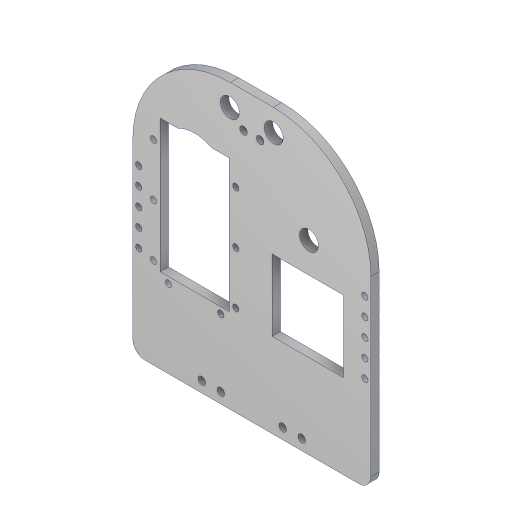
# Autodesk Inventor part: Box_Front
Saved by Autodesk Inventor 2023.2 (Build 272271000, 271)
## iProperties
Created: 2021-07-28
Part Number: Box_Front
Material: 알루미늄 6061
Document SubType Name: Modeling
Designer: user
Density: 2.7 g/cm^3
Appearance: 알루미늄 - 평지
Mass: 86.6795 g
Surface Area: 213.653 cm^2
Volume: 32.1035 cm^3
Author: user
Autodesk Inventor part; units mm, degrees
ref_plane "YZ Plane" through (0, 0, 0) normal (1, 0, 0) x (0, 1, 0)
ref_plane "XZ Plane" through (0, 0, 0) normal (0, 1, 0) x (-1, 0, 0)
ref_plane "XY Plane" through (0, 0, 0) normal (0, 0, 1) x (1, 0, 0)
sketch "스케치1" plane through (0, 0, 0) normal (0, 0, 1) x (1, 0, 0)
  line L0 (-50.01, 54) -> (50.01, 54)
  line L1 (50.01, 54) -> (50.01, -40)
  line L2 (50.01, -40) -> (-50.01, -40)
  line L3 (-50.01, -40) -> (-50.01, 54)
  point P0 (0, 0)
  dimension "d0" = 100.02
  dimension "d1" = 50.01
  dimension "d2" = 94
  dimension "d3" = 40
  constraints: 8 end point, 2 parallel, 1 horizontal, 1 perpendicular
  measures "d0" distance of L1.end L2.end
  measures "d1" distance from line of L3 point (0, 0)
  measures "d2" distance between parallel lines of L2 L0
  measures "d3" distance from line of L2 point (0, 0)
extrude "돌출1" add sketch "스케치1" along normal blind 3.5
sketch "스케치2" plane through (0, 0, 3.5) normal (0, 0, 1) x (1, 0, 0)
  circle A0 centre (-24.01, 13.1) radius 14
  line L0 (-50.01, -40) -> (50.01, -40) projected
  point P0 (0, 0)
  dimension "d6" = 28
  dimension "d7" = 24.01
  dimension "d8" = 53.1
  constraints: 1 centre point
  measures "d6" diameter of A0
  measures "d7" horizontal distance of point (0, 0) A0.centre
  measures "d8" distance from line of L0 A0.centre
extrude "돌출2" cut sketch "스케치2" against normal up to surface (3.5 mm away)
sketch "스케치3" plane through (0, 0, 3.5) normal (0, 0, 1) x (1, 0, 0)
  line L0 (-9.49, -29.6) -> (-38.53, -29.6)
  line L1 (-38.53, -29.6) -> (-38.53, 26.3)
  line L2 (-38.53, 26.3) -> (-9.49, 26.3)
  line L3 (-9.49, 26.3) -> (-9.49, -29.6)
  line L4 (-50.01, -40) -> (50.01, -40) projected
  circle A0 centre (-24.01, 13.1) radius 14 projected
  point P0 (0, 0)
  dimension "d11" = 10.4
  dimension "d12" = 55.9
  dimension "d13" = 29.04
  dimension "d14" = 14.52
  constraints: 8 end point, 2 parallel, 1 horizontal, 1 perpendicular
  measures "d11" distance between parallel lines of L4 L0
  measures "d12" distance between parallel lines of L0 L2
  measures "d13" distance between parallel lines of L3 L1
  measures "d14" distance from line of L1 A0.centre
extrude "돌출3" cut sketch "스케치3" against normal up to surface (3.5 mm away) contours L0 L1 L2 A0 L3 | A0 L2 picked at (-19.646, 17.031)
sketch "스케치4" plane through (0, 0, 3.5) normal (0, 0, 1) x (1, 0, 0)
  line L0 (-38.53, -29.6) -> (-38.53, 26.3) projected
  line L1 (-9.49, 26.3) -> (-9.49, -29.6) projected
  line L2 (-9.49, -29.6) -> (-38.53, -29.6) projected
  arc A0 (-19.3452, 26.3) -> (-28.6748, 26.3) centre (-24.01, 13.1) ccw projected
  arc A1 (-16.8854, 26.3) -> (-31.1346, 26.3) centre (-24.01, 13.1) ccw
  line L3 (-38.53, 26.3) -> (-28.6748, 26.3) projected
  line L4 (-19.3452, 26.3) -> (-9.49, 26.3) projected
  point P0 (0, 0)
  constraints: 2 point on circle, 2 point on line, 1 centre point, 1 coincident
extrude "돌출4" cut sketch "스케치4" against normal up to surface (3.5 mm away)
sketch "스케치5" plane through (0, 0, 3.5) normal (0, 0, 1) x (1, 0, 0)
  arc A0 (-16.8854, 26.3) -> (-31.1346, 26.3) centre (-24.01, 13.1) ccw projected
  circle A1 centre (-24.01, 13.1) radius 5
  circle A2 centre (-6.71, -4.9) radius 1.705
  circle A3 centre (-6.71, 17.1) radius 1.705
  circle A4 centre (-6.71, -26.9) radius 1.7
  circle A5 centre (-13.01, -32.2) radius 1.705
  circle A6 centre (-35.01, -32.2) radius 1.705
  circle A7 centre (-41.31, -26.9) radius 1.705
  circle A8 centre (-41.31, -4.9) radius 1.705
  circle A9 centre (-41.31, 17.1) radius 1.705
  circle A10 centre (-41.31, 17.1) radius 1.35
  circle A11 centre (-41.31, -4.9) radius 1.35
  circle A12 centre (-41.31, -26.9) radius 1.35
  circle A13 centre (-35.01, -32.2) radius 1.35
  circle A14 centre (-13.01, -32.2) radius 1.35
  circle A15 centre (-6.71, -26.9) radius 1.35
  circle A16 centre (-6.71, -4.9) radius 1.35
  circle A17 centre (-6.71, 17.1) radius 1.35
  point P0 (0, 0)
  dimension "d20" = 3.41
  dimension "d21" = 2.7
  dimension "d22" = 2.7
  dimension "d23" = 2.7
  dimension "d24" = 2.7
  dimension "d25" = 2.7
  dimension "d26" = 2.7
  dimension "d27" = 2.7
  dimension "d28" = 2.7
  constraints: 17 centre point, 8 coincident
  measures "d20" diameter of A9
  measures "d21" diameter of A10
  measures "d22" diameter of A11
  measures "d23" diameter of A12
  measures "d24" diameter of A13
  measures "d25" diameter of A14
  measures "d26" diameter of A15
  measures "d27" diameter of A16
  measures "d28" diameter of A17
extrude "돌출5" cut sketch "스케치5" against normal up to surface (3.5 mm away) contours A10 | A11 | A12 | A13 | A14 | A15 | A16 | A17
sketch "스케치6" plane through (0, 0, 3.5) normal (0, 0, 1) x (1, 0, 0)
  arc A0 (-16.8854, 26.3) -> (-31.1346, 26.3) centre (-24.01, 13.1) ccw projected
  line L0 (-24.01, 13.1) -> (24.01, 13.1)
  line L1 (-24.01, 13.1) -> (24.01, 13.1) construction
  circle A1 centre (24.01, 13.1) radius 4.025
  point P0 (0, 0)
  dimension "d31" = 48.02
  dimension "d32" = 0
  dimension "d33" = 8.05
  constraints: 4 end point, 2 horizontal, 1 centre point, 1 coincident, 1 collinear
  measures "d31" distance of L0.start L0.end
  measures "d32" distance between parallel lines of L0 L1
  measures "d33" diameter of A1
extrude "돌출6" cut sketch "스케치6" against normal up to surface (3.5 mm away)
chamfer "모따기2" distance 1.25 angle 45 8 edges at (-8.06, 17.1, 0) (-8.06, -4.9, 0) (-8.06, -26.9, 0) (-14.36, -32.2, 0) (-36.36, -32.2, 0) (-42.66, -26.9, 0) (-42.66, -4.9, 0) (-42.66, 17.1, 0)
sketch "스케치7" plane through (0, 0, 0) normal (0, 0, -1) x (-1, 0, 0)
  arc A0 (31.1346, 26.3) -> (16.8854, 26.3) centre (24.01, 13.1) ccw projected
  line L0 (24.01, 13.1) -> (9.2184, 44.8208)
  line L1 (24.01, 13.1) -> (59.01, 13.1) construction
  circle A1 centre (9.2184, 44.8208) radius 4.025
  circle A2 centre (-24.01, 13.1) radius 4.025 projected
  line L2 (-24.01, 13.1) -> (-9.2184, 44.8208)
  line L3 (-24.01, 13.1) -> (10.99, 13.1) construction
  circle A3 centre (-9.2184, 44.8208) radius 4.025
  point P0 (0, 0)
  dimension "d42" = 35
  dimension "d43" = 115
  dimension "d44" = 8.05
  dimension "d45" = 35
  dimension "d46" = 65
  dimension "d47" = 8.05
  constraints: 8 end point, 2 centre point, 2 coincident, 2 equal length, 2 horizontal
  measures "d42" distance of L0.start L0.end
  measures "d43" angle of L1 L0
  measures "d44" diameter of A1
  measures "d45" distance of L2.start L2.end
  measures "d46" angle of L3 L2
  measures "d47" diameter of A3
extrude "돌출7" cut sketch "스케치7" against normal up to surface (3.5 mm away) contours A1 | A3
fillet "모깎기1" radius 41 2 edges at (-50.01, 54, 1.75) (50.01, 54, 1.75)
sketch "스케치8" plane through (0, 0, 0) normal (0, 0, -1) x (-1, 0, 0)
  circle A0 centre (-47.51, -25.5) radius 1.35
  circle A1 centre (-47.51, -18) radius 1.35
  circle A2 centre (-47.51, -10.5) radius 1.35
  circle A3 centre (-47.51, -3) radius 1.35
  circle A4 centre (-47.51, 4.5) radius 1.35
  line L0 (-50.01, 13) -> (-50.01, -40) projected
  line L1 (-50.01, -40) -> (50.01, -40) projected
  point P0 (0, 0)
  dimension "d51" = 2.7
  dimension "d52" = 2.7
  dimension "d53" = 2.7
  dimension "d54" = 2.7
  dimension "d55" = 2.7
  dimension "d56" = 2.5
  dimension "d57" = 2.5
  dimension "d58" = 2.5
  dimension "d59" = 2.5
  dimension "d60" = 2.5
  dimension "d61" = 14.5
  dimension "d62" = 7.5
  dimension "d63" = 15
  dimension "d64" = 22.5
  dimension "d65" = 30
  constraints: 5 centre point
  measures "d51" diameter of A0
  measures "d52" diameter of A1
  measures "d53" diameter of A2
  measures "d54" diameter of A3
  measures "d55" diameter of A4
  measures "d56" distance from line of L0 A0.centre
  measures "d57" distance from line of L0 A1.centre
  measures "d58" distance from line of L0 A2.centre
  measures "d59" distance from line of L0 A3.centre
  measures "d60" distance from line of L0 A4.centre
  measures "d61" distance from line of A0.centre L1
  measures "d62" distance of A1.centre A0.centre
  measures "d63" distance of A2.centre A0.centre
  measures "d64" distance of A3.centre A0.centre
  measures "d65" distance of A4.centre A0.centre
extrude "돌출8" cut sketch "스케치8" against normal up to surface (3.5 mm away)
chamfer "모따기3" distance 1.25 angle 45 5 edges at (48.86, -25.5, 0) (48.86, -18, 0) (48.86, -10.5, 0) (48.86, -3, 0) (48.86, 4.5, 0)
sketch "스케치9" plane through (0, 0, 3.5) normal (0, 0, 1) x (1, 0, 0)
  circle A0 centre (-47.51, -25.5) radius 1.35
  circle A1 centre (-47.51, -18) radius 1.35
  circle A2 centre (-47.51, -10.5) radius 1.35
  circle A3 centre (-47.51, -3) radius 1.35
  circle A4 centre (-47.51, 4.5) radius 1.35
  line L0 (-50.01, 13) -> (-50.01, -40) projected
  line L1 (-50.01, -40) -> (50.01, -40) projected
  point P0 (0, 0)
  dimension "d71" = 2.7
  dimension "d72" = 2.7
  dimension "d73" = 2.7
  dimension "d74" = 2.7
  dimension "d75" = 2.7
  dimension "d76" = 2.5
  dimension "d77" = 2.5
  dimension "d78" = 2.5
  dimension "d79" = 2.5
  dimension "d80" = 2.5
  dimension "d81" = 14.5
  dimension "d82" = 22
  dimension "d83" = 29.5
  dimension "d84" = 37
  dimension "d85" = 44.5
  constraints: 5 centre point
  measures "d71" diameter of A0
  measures "d72" diameter of A1
  measures "d73" diameter of A2
  measures "d74" diameter of A3
  measures "d75" diameter of A4
  measures "d76" distance from line of L0 A4.centre
  measures "d77" distance from line of L0 A3.centre
  measures "d78" distance from line of L0 A2.centre
  measures "d79" distance from line of L0 A1.centre
  measures "d80" distance from line of L0 A0.centre
  measures "d81" distance from line of L1 A0.centre
  measures "d82" distance from line of L1 A1.centre
  measures "d83" distance from line of L1 A2.centre
  measures "d84" distance from line of L1 A3.centre
  measures "d85" distance from line of L1 A4.centre
extrude "돌출9" cut sketch "스케치9" against normal up to surface (3.5 mm away)
chamfer "모따기4" distance 1.25 angle 45 5 edges at (-48.86, 4.5, 0) (-48.86, -3, 0) (-48.86, -10.5, 0) (-48.86, -18, 0) (-48.86, -25.5, 0)
sketch "스케치10" plane through (0, 0, 0) normal (0, 0, -1) x (-1, 0, 0)
  line L0 (-50.01, -26.2141) -> (-50.01, -40) projected
  line L1 (50.01, -40) -> (50.01, -26.2141) projected
  line L2 (-50.01, -40) -> (50.01, -40) projected
  line L3 (-50.01, -40) -> (50.01, -40)
  line L4 (50.01, -40) -> (50.01, -65)
  line L5 (50.01, -65) -> (-50.01, -65)
  line L6 (-50.01, -65) -> (-50.01, -40)
  point P0 (0, 0)
  dimension "d100" = 25
  constraints: 8 end point, 2 parallel, 1 horizontal, 1 perpendicular
  measures "d100" distance of L3.end L4.end
extrude "돌출10" add sketch "스케치10" against normal up to surface (3.5 mm away)
sketch "스케치11" plane through (0, 0, 0) normal (0, 0, -1) x (-1, 0, 0)
  line L0 (-25, -58) -> (25, -58)
  line L1 (25, -58) -> (25, -63)
  line L2 (25, -63) -> (-25, -63)
  line L3 (-25, -63) -> (-25, -58)
  line L4 (50.01, -65) -> (-50.01, -65) projected
  circle A0 centre (-21, -60.5) radius 1.6
  circle A1 centre (-13, -60.5) radius 1.6
  circle A2 centre (13, -60.5) radius 1.6
  circle A3 centre (21, -60.5) radius 1.6
  point P0 (0, 0)
  dimension "d103" = 50
  dimension "d104" = 5
  dimension "d105" = 7
  dimension "d106" = 25
  dimension "d107" = 3.2
  dimension "d108" = 3.2
  dimension "d109" = 3.2
  dimension "d110" = 3.2
  dimension "d111" = 2.5
  dimension "d112" = 2.5
  dimension "d113" = 2.5
  dimension "d114" = 2.5
  dimension "d115" = 4
  dimension "d116" = 12
  dimension "d117" = 4
  dimension "d118" = 12
  constraints: 8 end point, 4 centre point, 2 parallel, 1 horizontal, 1 perpendicular
  measures "d103" distance of L1.end L2.end
  measures "d104" distance of L0.end L1.end
  measures "d105" distance between parallel lines of L4 L0
  measures "d106" distance from line of point (0, 0) L1
  measures "d107" diameter of A0
  measures "d108" diameter of A1
  measures "d109" diameter of A2
  measures "d110" diameter of A3
  measures "d111" distance from line of L2 A0.centre
  measures "d112" distance from line of L2 A1.centre
  measures "d113" distance from line of L2 A2.centre
  measures "d114" distance from line of L2 A3.centre
  measures "d115" distance from line of L3 A0.centre
  measures "d116" distance from line of L3 A1.centre
  measures "d117" distance from line of L1 A3.centre
  measures "d118" distance from line of L1 A2.centre
extrude "돌출11" cut sketch "스케치11" against normal up to surface (3.5 mm away) contours A0 | A1 | A2 | A3
fillet "모깎기2" radius 5 2 edges at (50.01, -65, 1.75) (-50.01, -65, 1.75)
sketch "스케치13" plane through (0, 0, 0) normal (0, 0, -1) x (-1, 0, 0)
  line L0 (9.49, 26.3) -> (16.8854, 26.3) projected
  line L1 (16.9, 29.3) -> (-16.9, 29.3)
  line L2 (16.9, 29.3) -> (50.7, 29.3) construction
  line L3 (9.01, 54) -> (-9.01, 54) projected
  line L4 (7, 36.3) -> (-7, 36.3)
  line L5 (-7, 36.3) -> (-7, 39.3)
  line L6 (-4, 42.3) -> (4, 42.3)
  line L7 (7, 39.3) -> (7, 36.3)
  circle A0 centre (3.5, 39.3) radius 1.6
  circle A1 centre (-3.5, 39.3) radius 1.6
  arc A2 (7, 39.3) -> (4, 42.3) centre (4, 39.3) ccw
  arc A3 (-4, 42.3) -> (-7, 39.3) centre (-4, 39.3) ccw
  point P0 (0, 0)
  point P1 (-7, 42.3)
  point P2 (7, 42.3)
  dimension "d149" = 33.8
  dimension "d150" = 180
  dimension "d151" = 16.9
  dimension "d153" = 14
  dimension "d154" = 6
  dimension "d155" = 13
  dimension "d156" = 7
  dimension "d157" = 3.2
  dimension "d158" = 3.2
  dimension "d159" = 3.5
  dimension "d160" = 3.5
  dimension "d161" = 3
  dimension "d162" = 3
  dimension "d169" = 3
  dimension "d170" = 3
  constraints: 12 end point, 4 centre point, 4 point on circle, 4 point on line, 4 tangent, 3 horizontal, 3 parallel, 1 collinear, 1 equal radius, 1 perpendicular
  measures "d149" distance of L1.start L1.end
  measures "d150" angle of L1 L2
  measures "d151" horizontal distance of L1.end point (0, 0)
  measures "d153" distance of point (-7, 42.3) point (7, 42.3)
  measures "d154" distance of L4.end point (-7, 42.3)
  measures "d155" distance between parallel lines of L6 L1
  measures "d156" distance from line of L7 point (0, 0)
  measures "d157" diameter of A0
  measures "d158" diameter of A1
  measures "d159" distance from line of L5 A1.centre
  measures "d160" distance from line of L7 A0.centre
  measures "d161" distance from line of L6 A0.centre
  measures "d162" distance from line of L6 A1.centre
  measures "d169" distance between parallel lines of L1 L0
  measures "d170" radius of A2
extrude "돌출13" cut sketch "스케치13" against normal up to surface (3.5 mm away) contours A0 | A1
chamfer "모따기6" distance 1.5 angle 45 2 edges at (-1.9, 39.3, 0) (5.1, 39.3, 0)
sketch "스케치17" plane through (0, 0, 0) normal (0, 0, -1) x (-1, 0, 0)
  line L0 (-8.51, 0.4) -> (-38.51, 0.4)
  line L1 (-38.51, 0.4) -> (-38.51, -29.6)
  line L2 (-38.51, -29.6) -> (-8.51, -29.6)
  line L3 (-8.51, -29.6) -> (-8.51, 0.4)
  line L4 (-8.51, 0.4) -> (-38.51, -29.6) construction
  line L5 (-38.51, 0.4) -> (-8.51, -29.6) construction
  line L6 (-50.01, -26.2141) -> (-50.01, -60) projected
  line L7 (45.01, -65) -> (-45.01, -65) projected
  point P0 (0, 0)
  point P1 (-23.51, -14.6)
  dimension "d182" = 30
  dimension "d183" = 30
  dimension "d185" = 35.4
  dimension "d188" = 11.5
  constraints: 12 end point, 2 midpoint, 2 parallel, 1 horizontal, 1 perpendicular
  measures "d182" distance of L2.end L1.end
  measures "d183" distance of L1.end L0.end
  measures "d185" distance between parallel lines of L7 L2
  measures "d188" distance between parallel lines of L6 L1
extrude "돌출17" cut sketch "스케치17" against normal blind 10
sketch "스케치15" plane through (0, 0, 0) normal (0, 0, -1) x (-1, 0, 0)
  circle A0 centre (-24.01, 13.1) radius 4.025 projected
  circle A1 centre (-24.01, 13.1) radius 4.8
  point P0 (0, 0)
  dimension "d175" = 9.6
  constraints: 1 centre point, 1 coincident
  measures "d175" diameter of A1
sketch "스케치16" plane through (0, 0, 0) normal (0, 0, -1) x (-1, 0, 0)
  circle A0 centre (9.2184, 44.8208) radius 4.025 projected
  circle A1 centre (-9.2184, 44.8208) radius 4.025 projected
  circle A2 centre (9.2184, 44.8208) radius 4.8
  circle A3 centre (-9.2184, 44.8208) radius 4.8
  point P0 (0, 0)
  dimension "d178" = 9.6
  dimension "d179" = 9.6
  constraints: 2 centre point, 2 coincident
  measures "d178" diameter of A2
  measures "d179" diameter of A3
equation "\"d1\" = 0.5 * d0"
equation "\"d14\" = 0.5 * d13"
equation "\"d106\" = 0.5 * d103"
equation "\"d151\" = 0.5 * d149"
equation "\"d156\" = 0.5 * d153"
